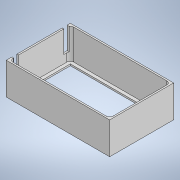
# Autodesk Inventor part: Крышка аккумулятора
Saved by Autodesk Inventor 2020 (Build 240168000, 168)
## iProperties
Created: 2021-08-09
Part Number: Крышка аккумулятора
Material: Типовые
Document SubType Name: Modeling
Designer: Антон
Density: 1 g/cm^3
Appearance: По умолчанию
Author: Антон
Autodesk Inventor part; units mm, degrees
ref_plane "YZ Plane" through (0, 0, 0) normal (1, 0, 0) x (0, 1, 0)
ref_plane "XZ Plane" through (0, 0, 0) normal (0, 1, 0) x (-1, 0, 0)
ref_plane "XY Plane" through (0, 0, 0) normal (0, 0, 1) x (1, 0, 0)
sketch "Эскиз1" plane through (0, 0, 0) normal (0, 1, 0) x (-1, 0, 0)
  line L0 (0, 0) -> (63.1, 0)
  line L1 (63.1, 0) -> (63.1, -39.1)
  line L2 (63.1, -39.1) -> (0, -39.1)
  line L3 (0, -39.1) -> (0, 0)
  dimension "d0" = 63.1
  dimension "d1" = 39.1
  constraints: 8 end point, 2 parallel, 1 horizontal, 1 perpendicular
  measures "d0" distance of L1.end L2.end
  measures "d1" distance of L0.end L1.end
extrude "Выдавливание1" add sketch "Эскиз1" along normal blind 19.5
shell "Оболочка1" thickness 1 removed faces 1 at (-42.0667, 19.5, -26.0667)
sketch "Эскиз2" plane through (0, 19.5, 0) normal (0, 1, 0) x (1, 0, 0)
  line L0 (-62.1, 38.1) -> (-62.1, 1) projected
  line L1 (-63.1, 39.1) -> (-63.1, 0) projected
  line L2 (-62.1, 37.1) -> (-63.1, 37.1)
  line L3 (-63.1, 37.1) -> (-63.1, 34.1)
  line L4 (-63.1, 34.1) -> (-62.1, 34.1)
  line L5 (-62.1, 3.5) -> (-63.1, 3.5)
  line L6 (-63.1, 3.5) -> (-63.1, 6.5)
  line L7 (-63.1, 6.5) -> (-62.1, 6.5)
  line L8 (-62.1, 38.1) -> (-1, 38.1) projected
  line L9 (-62.1, 34.1) -> (-62.1, 37.1)
  line L10 (-62.1, 6.5) -> (-62.1, 3.5)
  line L11 (-62.1, 1) -> (-62.1, 38.1) projected
  line L12 (-1, 1) -> (-62.1, 1) projected
  point P0 (0, 0)
  point P1 (-63.1, 35.6)
  point P2 (-63.1, 5)
  dimension "d5" = 3
  dimension "d11" = 2.5
  dimension "d12" = 3
  dimension "d13" = 4
  constraints: 16 end point, 3 collinear, 3 parallel, 2 horizontal, 2 midpoint, 2 perpendicular, 2 point on line
  measures "d5" distance of L3.end L2.end
  measures "d11" distance from line of L8 point (-63.1, 35.6)
  measures "d12" distance of L5.end L6.end
  measures "d13" distance from line of L12 point (-63.1, 5)
extrude "Выдавливание2" cut sketch "Эскиз2" against normal blind 13.5 contours L0 L4 L1 L2 | L0 L5 L1 L7
fillet "Сопряжение1" radius 2.15 4 edges at (-1, 10.25, -38.1) (-1, 10.25, -1) (-62.1, 10.25, -38.1) (-62.1, 10.25, -1)
sketch "Эскиз4" plane through (-62.1, 1, -1) normal (0, 1, 0) x (1, 0, 0)
  line L0 (0, 37.1) -> (0, 0) construction
  line L1 (61.1, 0) -> (0, 0) construction
  line L2 (0, 37.1) -> (61.1, 0) construction
  line L3 (2, 2) -> (59.1, 2)
  line L4 (59.1, 2) -> (59.1, 35.1)
  line L5 (59.1, 35.1) -> (2, 35.1)
  line L6 (2, 35.1) -> (2, 2)
  line L7 (2, 2) -> (59.1, 35.1) construction
  line L8 (59.1, 2) -> (2, 35.1) construction
  line L9 (30.55, 35.1) -> (30.55, 37.1) construction
  line L10 (0, 37.1) -> (61.1, 37.1) construction
  line L11 (59.1, 18.55) -> (61.1, 18.55) construction
  line L12 (61.1, 0) -> (61.1, 37.1) construction
  point P0 (62.1, -1)
  point P1 (-1.5, 0)
  point P2 (30.55, 18.55)
  point P3 (-1.5, 36.1)
  dimension "d8" = 2
  constraints: 18 end point, 6 midpoint, 2 parallel, 2 perpendicular, 1 horizontal, 1 vertical, 2 other
  measures "d8" distance of L9.start L9.end
extrude "Выдавливание3" cut sketch "Эскиз4" against normal through all
